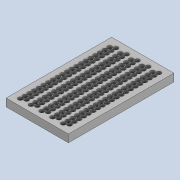
# Autodesk Inventor part: Model_Sita
Saved by Autodesk Inventor 2021.3 (Build 253353000, 353)
## iProperties
Created: 2023-05-23
Part Number: Model_Sita
Material: Ogólny
Document SubType Name: Modeling
Designer: User
Density: 1 g/cm^3
Appearance: Gładki — średnioszary
Author: User
Autodesk Inventor part; units mm, degrees
ref_plane "YZ Plane" through (0, 0, 0) normal (1, 0, 0) x (0, 1, 0)
sketch "Szkic1" plane through (0, 0, 0) normal (0, 1, 0) x (-1, 0, 0)
  line L0 (325, 550) -> (-325, 550)
  line L1 (-325, 550) -> (-325, -550)
  line L2 (-325, -550) -> (325, -550)
  line L3 (325, -550) -> (325, 550)
  point P0 (0, 0)
  point P1 (0, -550)
  point P2 (325, 0)
  dimension "d2" = 1100
  dimension "d3" = 650
  constraints: 8 end point, 2 midpoint, 2 parallel, 1 horizontal, 1 horizontal alignment, 1 perpendicular, 1 vertical alignment
  measures "d2" distance of L2.end L0.start
  measures "d3" distance of L0.start L0.end
extrude "Wyciągnięcie proste1" add sketch "Szkic1" along normal blind 80
sketch "Szkic3" plane through (0, 80, 0) normal (0, 1, 0) x (1, 0, 0)
  circle A0 centre (-245, -482) radius 23
  line L0 (-325, 550) -> (-325, -550) projected
  line L1 (-325, -550) -> (325, -550) projected
  circle A1 centre (-203, -458) radius 23
  point P0 (0, 0)
  dimension "d17" = 46
  dimension "d18" = 80
  dimension "d19" = 68
  dimension "d25" = 46
  dimension "d27" = 24
  dimension "d28" = 42
  constraints: 2 centre point
  measures "d17" diameter of A0
  measures "d18" distance from line of L0 A0.centre
  measures "d19" distance from line of L1 A0.centre
  measures "d25" diameter of A1
  measures "d27" vertical distance of A1.centre A0.centre
  measures "d28" horizontal distance of A0.centre A1.centre
extrude "Wyciągnięcie proste2" cut sketch "Szkic3" against normal blind 80
pattern_linear "Szyk prostokątny1" count 20 spacing 49 along (0, 0, -1) of "Wyciągnięcie proste2"
pattern_linear "Szyk prostokątny2" count 5 spacing 112 along (1, 0, 0) of "Wyciągnięcie proste2", "Szyk prostokątny1"
sketch "Szkic5" plane through (0, 80, 0) normal (0, 1, 0) x (1, 0, 0)
  line L0 (-281, -473) -> (-281, 550)
  line L1 (325, 550) -> (-325, 550) projected
  line L2 (-167, 464) -> (-167, -473)
  line L3 (-56, 464) -> (-56, -473)
  circle A0 centre (-91, -17) radius 23 projected
  circle A1 centre (-203, -17) radius 23 projected
  circle A2 centre (-245, -41) radius 23 projected
  circle A3 centre (-245, -482) radius 23 projected
  circle A4 centre (-133, 449) radius 23 projected
  line L4 (-117, 514) -> (-106, 514)
  arc A5 (-117, 514) -> (-167, 464) centre (-117, 464) ccw
  arc A6 (-56, 464) -> (-106, 514) centre (-106, 464) ccw
  line L5 (-231, -523) -> (-217, -523)
  arc A7 (-281, -473) -> (-231, -523) centre (-231, -473) ccw
  arc A8 (-217, -523) -> (-167, -473) centre (-217, -473) ccw
  circle A9 centre (-203, -458) radius 23 projected
  circle A10 centre (21, -360) radius 23 projected
  arc A11 (-56, -473) -> (0.172, -527.9875) centre (-1, -473) ccw
  circle A12 centre (21, -458) radius 23 projected
  point P0 (0, 0)
  point P1 (-281, -523)
  point P2 (-56, 514)
  dimension "d34" = 35
  dimension "d35" = 36
  dimension "d36" = 36
  dimension "d48" = 50
  dimension "d49" = 50
  dimension "d50" = 15
  dimension "d51" = 50
  dimension "d54" = 15
  dimension "d56" = 55
  dimension "d57" = 15
  constraints: 10 end point, 10 point on circle, 9 tangent, 5 centre point, 5 point on line, 3 vertical, 2 horizontal, 1 equal radius
  measures "d34" distance from line of A0.centre L3
  measures "d35" distance from line of A1.centre L2
  measures "d36" distance from line of A2.centre L0
  measures "d48" radius of A5
  measures "d49" radius of A6
  measures "d50" vertical distance of A4.centre A5.centre
  measures "d51" radius of A7
  measures "d54" vertical distance of A9.centre A8.centre
  measures "d56" radius of A11
  measures "d57" vertical distance of A12.centre A11.centre
ref_plane "Płaszczyzna konstrukcyjna1" through (-281, 80, -550) normal (0, 0, -1) x (-1, 0, 0)
sketch "Szkic6" plane through (-281, 80, -550) normal (0, 0, -1) x (-1, 0, 0)
  line L0 (-5, -5.4895) -> (5, -5.4895)
  line L1 (5, -5.4895) -> (5, -75.4895)
  line L2 (5, -75.4895) -> (-5, -75.4895)
  line L3 (-5, -75.4895) -> (-5, -5.4895)
  point P0 (-281, -80)
  point P1 (0, 0)
  dimension "d41" = 5
  dimension "d42" = 5
  dimension "d43" = 70
  constraints: 8 end point, 2 parallel, 1 horizontal, 1 perpendicular
  measures "d41" distance from line of L1 point (0, 0)
  measures "d42" distance from line of point (0, 0) L3
  measures "d43" distance between parallel lines of L2 L0
sweep "Przeciągnięcie1" cut profiles "Szkic6" path "Szkic5" path curves L0 A7 L5 A8 L2 A5 L4 A6 L3 A11
ref_plane "Płaszczyzna konstrukcyjna2" through (0, 0, 550) normal (1, 0, 0) x (0, 0, -1)
mirror "Odbij2" about plane through (0, 0, 550) normal (1, 0, 0) of "Przeciągnięcie1"
equation "\"d24\" = Odleglosc_od_sr_ogniw"
equation "\"Odleglosc_od_sr_ogniw\" = 49"
